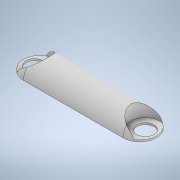
# Autodesk Inventor part: Retention Clip - Whisper Valve Horizontal
Saved by Autodesk Inventor 2020 (Build 240168000, 168)
## iProperties
Created: 2022-06-20
Part Number: Retention Clip - Whisper Valve Horizontal
Material: Generic
Document SubType Name: Modeling
Designer: Beaucage
Density: 1 g/cm^3
Appearance: Default
Author: Beaucage
Autodesk Inventor part; units mm, degrees
ref_plane "YZ Plane" through (0, 0, 0) normal (1, 0, 0) x (0, 1, 0)
ref_plane "XZ Plane" through (0, 0, 0) normal (0, 1, 0) x (-1, 0, 0)
ref_plane "XY Plane" through (0, 0, 0) normal (0, 0, 1) x (1, 0, 0)
sketch "Sketch1" plane through (0, 0, 0) normal (0, 1, 0) x (-1, 0, 0)
  line L0 (0, 0) -> (25.4, 0)
  line L1 (25.4, 0) -> (25.4, -6.35)
  line L2 (25.4, -6.35) -> (0, -6.35)
  line L3 (0, -6.35) -> (0, 0)
  dimension "d0" = 25.4
  dimension "d1" = 6.35
  constraints: 8 end point, 2 parallel, 1 horizontal, 1 perpendicular
  measures "d0" distance of L1.end L2.end
  measures "d1" distance of L0.end L1.end
extrude "Extrusion1" add sketch "Sketch1" along normal blind 3.175
sketch "Sketch2" plane through (0, 3.175, 0) normal (0, 1, 0) x (1, 0, 0)
  line L0 (0, 0) -> (0, 6.35) projected
  line L1 (0, 3.175) -> (-2.1082, 3.175)
  line L2 (-25.4, 6.35) -> (-25.4, 0) projected
  line L3 (-25.4, 3.175) -> (-23.2918, 3.175)
  dimension "d4" = 2.1082
  dimension "d5" = 2.1082
  constraints: 4 end point, 2 horizontal, 2 midpoint
  measures "d4" distance of L1.start L1.end
  measures "d5" distance of L3.start L3.end
hole "Hole1" at (-23.2918, 3.175, -3.175) at (-2.1082, 3.175, -3.175) direction (0, -1, 0) diameter 3.2766 depth 5.6896 counterbore diameter 5.5626 counterbore depth 2.8448 clearance for "Socket Head Cap Screw" size "#4" standard "Ansi Unified Screw Threads"
fillet "Fillet1" radius 3.175 6 edges at (-12.7, 3.175, 0) (-12.7, 3.175, -6.35) (-25.4, 3.175, -5.6696) (-25.4, 3.175, -0.6804) (0, 3.175, -5.6696) (0, 3.175, -0.6804)
fillet "Fillet2" radius 3.175 4 edges at (0, 1.4698, -5.9893) (0, 1.4698, -0.3607) (-25.4, 1.4698, -5.9893) (-25.4, 1.4698, -0.3607)
body "Solid1"
